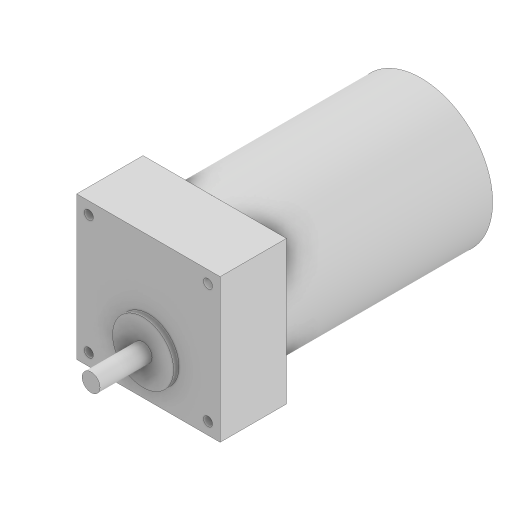
# Autodesk Inventor part: MOTOR DC
Saved by Autodesk Inventor 2024 (Build 280153000, 153)
## iProperties
Created: 2024-05-26
Part Number: MOTOR DC
Material: Generic
Document SubType Name: Modeling
Designer: Jhuliams
Density: 1 g/cm^3
Appearance: Default
Author: Jhuliams
Autodesk Inventor part; units mm, degrees
ref_plane "YZ Plane" through (0, 0, 0) normal (1, 0, 0) x (0, 1, 0)
ref_plane "XZ Plane" through (0, 0, 0) normal (0, 1, 0) x (-1, 0, 0)
ref_plane "XY Plane" through (0, 0, 0) normal (0, 0, 1) x (1, 0, 0)
sketch "Sketch1" plane through (0, 0, 0) normal (0, 0, 1) x (1, 0, 0)
  circle A0 centre (0, 0) radius 40
  dimension "d0" = 80
  constraints: 1 centre point, 1 coincident
  measures "d0" diameter of A0
extrude "Extrusion1" add sketch "Sketch1" along normal mid plane 115
sketch "Sketch3" plane through (0, 0, 57.5) normal (0, 0, 1) x (1, 0, 0)
  line L0 (-40, 40) -> (40, 40)
  line L1 (40, 40) -> (40, -40)
  line L2 (40, -40) -> (-40, -40)
  line L3 (-40, -40) -> (-40, 40)
  line L4 (-40, 40) -> (40, -40) construction
  line L5 (40, 40) -> (-40, -40) construction
  point P0 (0, 0)
  dimension "d9" = 80
  dimension "d10" = 80
  constraints: 12 end point, 2 parallel, 1 horizontal, 1 perpendicular
  measures "d9" distance of L1.end L2.end
  measures "d10" distance of L0.end L1.end
extrude "Extrusion3" add sketch "Sketch3" along normal blind 37
sketch "Sketch4" plane through (0, 0, 94.5) normal (0, 0, 1) x (1, 0, 0)
  line L0 (0, 0) -> (0, -15)
  circle A0 centre (0, -15) radius 5
  dimension "d11" = 15
  dimension "d12" = 10
  constraints: 2 end point, 1 centre point, 1 coincident, 1 vertical
  measures "d11" distance of L0.start L0.end
  measures "d12" diameter of A0
extrude "Extrusion4" add sketch "Sketch4" along normal blind 32
sketch "Sketch5" plane through (0, 0, 94.5) normal (0, 0, 1) x (1, 0, 0)
  circle A0 centre (0, -15) radius 17
  point P0 (0, 0)
  dimension "d15" = 34
  constraints: 1 centre point
  measures "d15" diameter of A0
extrude "Extrusion5" add sketch "Sketch5" along normal blind 3
sketch "Sketch6" plane through (0, 0, 94.5) normal (0, 0, 1) x (1, 0, 0)
  circle A0 centre (0, 0) radius 47
  line L0 (40, 0) -> (40, 40) projected
  line L1 (-40, 0) -> (-40, -40) projected
  line L2 (40, 40) -> (-40, -40)
  line L3 (-40, -40) -> (-40, 40)
  line L4 (40, -40) -> (40, 40) projected
  line L5 (-40, 40) -> (40, -40)
  circle A1 centre (33.234, 33.234) radius 2.5
  circle A2 centre (-33.234, 33.234) radius 2.5
  circle A3 centre (-33.234, -33.234) radius 2.5
  circle A4 centre (33.234, -33.234) radius 2.5
  dimension "d18" = 94
  dimension "d19" = 5
  dimension "d22" = 360
  constraints: 6 end point, 4 centre point, 1 coincident, 1 collinear, 1 perpendicular, 1 point on line, 12 other
  measures "d19" diameter of A1
extrude "Extrusion6" cut sketch "Sketch6" against normal blind 40 contours A1 L2 A0 | A0 L2 A1 | A4 L5 A0 | A0 L5 A4 | L2 A1 A0 | A0 A1 L2 | L5 A4 A0 | A0 A4 L5 | A2 L5 A0 | A0 L5 A2 | A3 A0 L2 | L2 A0 A3 | A2 A0 L5 | A3 L2 A0 | A0 A2 L5 | L2 A3 A0
body "Solid1"
